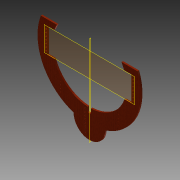
# Autodesk Inventor part: gyroYoke01_resized01
Saved by Autodesk Inventor 2013 (Build 170138000, 138)
## iProperties
Created: 2013-02-24
Part Number: gyroYoke01_resized01
Material: Wood (Oak)
Document SubType Name: Modeling
Designer: Nano
Density: 0.56 g/cm^3
Mass: 146.727 g
Surface Area: 937.732 cm^2
Volume: 262.012 cm^3
d0: 0.125 in
d1: 1.000 in
d3: 0.250 in
d4: 0.00 deg
d5: 0.250 in
d6: 0.250 in
d7: 0.250 in
d8: 0.250 in
d9: 0.125 in
d10: 0.125 in
d11: 0.250 in
d13: 0.250 in
d14: 0.00 deg
d15: 0.125 in
d22: 6.000 ul
d24: 0.500 in
d26: 0.00 deg
d27: 0.125 in
d34: 6.000 ul
d36: 0.500 in
d12: 0.250 in
Author: Nano
Autodesk Inventor part; units mm, degrees
ref_plane "YZ Plane" through (0, 0, 0) normal (1, 0, 0) x (0, 1, 0)
ref_plane "XZ Plane" through (0, 0, 0) normal (0, 1, 0) x (-1, 0, 0)
ref_plane "XY Plane" through (0, 0, 0) normal (0, 0, 1) x (1, 0, 0)
ref_plane "Work Plane1" through (0, 0, 0) normal (0, 0, 1) x (1, 0, 0)
sketch "Sketch1" plane through (0, 0, 0) normal (0, 0, 1) x (1, 0, 0)
  circle A0 centre (166.6875, 44.45) radius 6.35 construction
  line L0 (0, 0) -> (333.375, 0) construction
  line L1 (333.375, 0) -> (333.375, 88.9) construction
  line L2 (0, 88.9) -> (333.375, 88.9) construction
  line L3 (0, 0) -> (0, 88.9) construction
  line L4 (336.55, 95.25) -> (336.55, -6.35)
  line L5 (-3.175, -6.35) -> (-3.175, 95.25)
  arc A1 (361.952, -28.5758) -> (361.6406, 118.3031) centre (166.6875, 44.45) ccw
  arc A2 (109.447, -157.0949) -> (223.6431, -156.0919) centre (166.5241, -154.21) ccw
  arc A3 (223.6431, -156.0919) -> (230.1571, -154.1264) centre (166.6875, 44.45) ccw
  arc A4 (-29.5537, -28.941) -> (103.1936, -155.2131) centre (166.6875, 44.45) ccw
  arc A5 (-29.5402, 117.8769) -> (-29.5537, -28.941) centre (166.6875, 44.45) ccw
  arc A6 (336.55, 165.3087) -> (333.375, 169.6513) centre (166.6875, 44.45) ccw
  arc A7 (0, 169.6513) -> (-3.175, 165.3087) centre (166.6875, 44.45) ccw
  line L6 (361.6406, 118.3031) -> (296.5092, 118.3031)
  line L7 (35.5855, 117.8769) -> (-29.5402, 117.8769)
  arc A8 (194.8672, -103.8723) -> (308.8598, -6.35) centre (166.6875, 44.45) ccw
  arc A9 (307.1415, 95.25) -> (296.5092, 118.3031) centre (166.6875, 44.45) ccw
  arc A10 (35.5855, 117.8769) -> (25.271, 95.25) centre (166.6875, 44.45) ccw
  arc A11 (24.5152, -6.35) -> (136.5493, -103.4867) centre (166.6875, 44.45) ccw
  line L8 (-3.175, 95.25) -> (25.271, 95.25)
  line L9 (307.1415, 95.25) -> (336.55, 95.25)
  line L10 (336.55, -6.35) -> (308.8598, -6.35)
  line L11 (24.5152, -6.35) -> (-3.175, -6.35)
  line L12 (173.0375, -106.3919) -> (173.0375, -125.2673)
  line L13 (173.0375, -125.2673) -> (160.3375, -125.2673)
  line L14 (160.3375, -125.2673) -> (160.3375, -106.3919)
  line L15 (163.5125, -117.9837) -> (169.8625, -117.9837) projected
  line L16 (166.6875, 44.45) -> (38.9307, -83.3068) projected
  arc A12 (136.5493, -103.4867) -> (160.3375, -106.3919) centre (166.6875, 44.45) ccw
  arc A13 (173.0375, -106.3919) -> (194.8672, -103.8723) centre (166.6875, 44.45) ccw
  arc A14 (230.1571, -154.1264) -> (103.1936, -155.2131) centre (166.6875, -156.0919) ccw
  arc A15 (230.1571, -154.1264) -> (361.952, -28.5758) centre (166.6875, 44.45) ccw
  arc A16 (103.1936, -155.2131) -> (109.447, -157.0949) centre (166.6875, 44.45) ccw
  arc A17 (103.1936, -155.2131) -> (230.1571, -154.1264) centre (166.6875, -156.0919) ccw
  point P0 (166.6875, -117.9837)
  dimension "d0" = 3.175
  dimension "d5" = 6.35
  dimension "d6" = 6.35
  dimension "d7" = 6.35
  dimension "d8" = 6.35
  dimension "d9" = 3.175
  dimension "d10" = 3.175
  dimension "d11" = 6.35
  dimension "d12" = 6.35
  dimension "d47" = 127
  constraints: 34 point on circle, 22 end point, 17 centre point, 4 point on line, 1 coincident, 1 parallel, 1 other
  measures "d0" distance between parallel lines of L4 L1
  measures "d5" distance between parallel lines of L2 L9
  measures "d6" distance between parallel lines of L0 L10
  measures "d7" distance between parallel lines of L2 L8
  measures "d8" distance between parallel lines of L0 L11
  measures "d9" distance from line of L14 L15.start
  measures "d10" distance from line of L15.end L12
  measures "d11" distance from line of L12 point (166.688, -117.984)
  measures "d12" distance from line of point (166.688, -117.984) L14
  measures "d47" diameter of A14
extrude "Extrusion1" add sketch "Sketch1" against normal blind 6.35 contours L9 A9 L6 A1 A15 A14 A8 L10 L4 | A14 A3 A2 A16 A11 A12 L14 L13 L12 A13 A8 | A17 A16 A2 A3 | A14 A4 A5 L7 A10 L8 L5 L11 A11
sketch "Sketch2" plane through (0, 0, 0) normal (0, 0, 1) x (1, 0, 0)
  line L0 (339.725, 79.375) -> (346.075, 79.375) projected
  line L1 (346.075, 85.725) -> (346.075, 79.375) projected
  line L2 (346.075, 85.725) -> (339.725, 85.725) projected
  line L3 (339.725, 85.725) -> (339.725, 79.375) projected
  line L4 (339.725, 66.675) -> (346.075, 66.675) projected
  line L5 (346.075, 73.025) -> (346.075, 66.675) projected
  line L6 (346.075, 73.025) -> (339.725, 73.025) projected
  line L7 (339.725, 73.025) -> (339.725, 66.675) projected
  line L8 (339.725, 53.975) -> (346.075, 53.975) projected
  line L9 (346.075, 60.325) -> (346.075, 53.975) projected
  line L10 (346.075, 60.325) -> (339.725, 60.325) projected
  line L11 (339.725, 60.325) -> (339.725, 53.975) projected
  line L12 (346.075, 47.625) -> (339.725, 47.625) projected
  line L13 (339.725, 47.625) -> (339.725, 41.275) projected
  line L14 (339.725, 41.275) -> (346.075, 41.275) projected
  line L15 (346.075, 47.625) -> (346.075, 41.275) projected
  line L16 (346.075, 34.925) -> (339.725, 34.925) projected
  line L17 (339.725, 34.925) -> (339.725, 28.575) projected
  line L18 (339.725, 28.575) -> (346.075, 28.575) projected
  line L19 (346.075, 34.925) -> (346.075, 28.575) projected
  line L20 (346.075, 22.225) -> (339.725, 22.225) projected
  line L21 (339.725, 22.225) -> (339.725, 15.875) projected
  line L22 (339.725, 15.875) -> (346.075, 15.875) projected
  line L23 (346.075, 22.225) -> (346.075, 15.875) projected
  line L24 (346.075, 9.525) -> (339.725, 9.525) projected
  line L25 (339.725, 9.525) -> (339.725, 3.175) projected
  line L26 (339.725, 3.175) -> (346.075, 3.175) projected
  line L27 (346.075, 9.525) -> (346.075, 3.175) projected
  point P0 (0, 0)
extrude "Extrusion2" cut sketch "Sketch2" against normal blind 6.35
sketch "Sketch3" plane through (0, 0, 0) normal (0, 0, 1) x (1, 0, 0)
  line L0 (339.725, 15.875) -> (346.075, 9.525) construction
  line L1 (346.075, 15.875) -> (339.725, 9.525) construction
  point P0 (0, 0)
  point P1 (342.9, 12.7)
  constraints: 4 end point
hole "Hole1" at (342.9, 12.7, 0) direction (0, 0, -1) diameter 3.175 end through all
pattern_linear "Rectangular Pattern1" count 6 spacing 12.7 along (0, 1, 0) of "Hole1"
ref_plane "Work Plane2" through (166.6875, -125.2673, 0) normal (1, 0, 0) x (0, 0, -1)
mirror "Mirror1" about plane through (166.6875, -125.2673, 0) normal (1, 0, 0) of "Extrusion2", "Hole1", "Rectangular Pattern1"
sketch "Sketch5" plane through (0, 0, 0) normal (0, 0, 1) x (1, 0, 0)
  line L0 (150.8125, -110.6581) -> (147.6375, -110.6581)
  line L1 (147.6375, -110.6581) -> (147.6375, -116.7384)
  line L2 (147.6375, -116.7384) -> (150.8125, -116.7384)
  line L3 (150.8125, -110.6581) -> (150.8125, -116.7384)
  line L4 (147.6375, -129.4384) -> (150.8125, -129.4384)
  line L5 (150.8125, -123.0884) -> (150.8125, -129.4384)
  line L6 (150.8125, -123.0884) -> (147.6375, -123.0884)
  line L7 (147.6375, -123.0884) -> (147.6375, -129.4384)
  line L8 (150.8125, -135.7884) -> (147.6375, -135.7884)
  line L9 (147.6375, -135.7884) -> (147.6375, -142.1384)
  line L10 (147.6375, -142.1384) -> (150.8125, -142.1384)
  line L11 (150.8125, -135.7884) -> (150.8125, -142.1384)
  line L12 (147.6375, -154.8384) -> (150.8125, -154.8384)
  line L13 (150.8125, -148.4884) -> (150.8125, -154.8384)
  line L14 (150.8125, -148.4884) -> (147.6375, -148.4884)
  line L15 (147.6375, -148.4884) -> (147.6375, -154.8384)
  line L16 (150.8125, -161.1884) -> (147.6375, -161.1884)
  line L17 (147.6375, -161.1884) -> (147.6375, -167.5384)
  line L18 (147.6375, -167.5384) -> (150.8125, -167.5384)
  line L19 (150.8125, -161.1884) -> (150.8125, -167.5384)
  line L20 (147.6375, -180.2384) -> (150.8125, -180.2384)
  line L21 (150.8125, -173.8884) -> (150.8125, -180.2384)
  line L22 (150.8125, -173.8884) -> (147.6375, -173.8884)
  line L23 (147.6375, -173.8884) -> (147.6375, -180.2384)
  line L24 (150.8125, -186.5884) -> (147.6375, -186.5884)
  line L25 (147.6375, -186.5884) -> (147.6375, -202.4634)
  line L26 (147.6375, -202.4634) -> (150.8125, -202.4634)
  line L27 (150.8125, -186.5884) -> (150.8125, -202.4634)
  point P0 (0, 0)
extrude "Extrusion3" cut sketch "Sketch5" against normal through all
sketch "Sketch6" plane through (0, 0, 0) normal (0, 0, 1) x (1, 0, 0)
  line L0 (150.8125, -173.8884) -> (150.8125, -180.2384) construction
  line L1 (150.8125, -180.2384) -> (147.6375, -180.2384) construction
  line L2 (147.6375, -180.2384) -> (147.6375, -173.8884) construction
  line L3 (147.6375, -173.8884) -> (150.8125, -173.8884) construction
  line L4 (150.8125, -148.4884) -> (150.8125, -154.8384) construction
  line L5 (150.8125, -154.8384) -> (147.6375, -154.8384) construction
  line L6 (147.6375, -154.8384) -> (147.6375, -148.4884) construction
  line L7 (147.6375, -148.4884) -> (150.8125, -148.4884) construction
  line L8 (150.8125, -123.0884) -> (150.8125, -129.4384) construction
  line L9 (150.8125, -129.4384) -> (147.6375, -129.4384) construction
  line L10 (147.6375, -129.4384) -> (147.6375, -123.0884) construction
  line L11 (147.6375, -123.0884) -> (150.8125, -123.0884) construction
  line L12 (147.6375, -116.7384) -> (147.6375, -110.6581) construction
  line L13 (147.6375, -110.6581) -> (150.8125, -110.6581) construction
  line L14 (150.8125, -110.6581) -> (150.8125, -116.7384) construction
  line L15 (150.8125, -116.7384) -> (147.6375, -116.7384) construction
  line L16 (147.6375, -142.1384) -> (147.6375, -135.7884) construction
  line L17 (147.6375, -135.7884) -> (150.8125, -135.7884) construction
  line L18 (150.8125, -135.7884) -> (150.8125, -142.1384) construction
  line L19 (150.8125, -142.1384) -> (147.6375, -142.1384) construction
  line L20 (147.6375, -167.5384) -> (147.6375, -161.1884) construction
  line L21 (147.6375, -161.1884) -> (150.8125, -161.1884) construction
  line L22 (150.8125, -161.1884) -> (150.8125, -167.5384) construction
  line L23 (150.8125, -167.5384) -> (147.6375, -167.5384) construction
  line L24 (147.6375, -202.4634) -> (147.6375, -186.5884) construction
  line L25 (147.6375, -186.5884) -> (150.8125, -186.5884) construction
  line L26 (150.8125, -186.5884) -> (150.8125, -202.4634) construction
  line L27 (150.8125, -202.4634) -> (147.6375, -202.4634) construction
  circle A0 centre (-9.525, 76.2) radius 1.5875 construction
  circle A1 centre (-9.525, 63.5) radius 1.5875 construction
  circle A2 centre (-9.525, 50.8) radius 1.5875 construction
  circle A3 centre (-9.525, 38.1) radius 1.5875 construction
  circle A4 centre (-9.525, 25.4) radius 1.5875 construction
  line L28 (-6.35, 9.525) -> (-6.35, 3.175) construction
  line L29 (-6.35, 3.175) -> (-12.7, 3.175) construction
  line L30 (-12.7, 3.175) -> (-12.7, 9.525) construction
  line L31 (-12.7, 9.525) -> (-6.35, 9.525) construction
  line L32 (-6.35, 34.925) -> (-6.35, 28.575) construction
  line L33 (-6.35, 28.575) -> (-12.7, 28.575) construction
  line L34 (-12.7, 28.575) -> (-12.7, 34.925) construction
  line L35 (-12.7, 34.925) -> (-6.35, 34.925) construction
  line L36 (-12.7, 53.975) -> (-12.7, 60.325) construction
  line L37 (-12.7, 60.325) -> (-6.35, 60.325) construction
  line L38 (-6.35, 60.325) -> (-6.35, 53.975) construction
  line L39 (-6.35, 53.975) -> (-12.7, 53.975) construction
  line L40 (-12.7, 79.375) -> (-12.7, 85.725) construction
  line L41 (-12.7, 85.725) -> (-6.35, 85.725) construction
  line L42 (-6.35, 85.725) -> (-6.35, 79.375) construction
  line L43 (-6.35, 79.375) -> (-12.7, 79.375) construction
  line L44 (-12.7, 66.675) -> (-12.7, 73.025) construction
  line L45 (-12.7, 73.025) -> (-6.35, 73.025) construction
  line L46 (-6.35, 73.025) -> (-6.35, 66.675) construction
  line L47 (-6.35, 66.675) -> (-12.7, 66.675) construction
  line L48 (-6.35, 47.625) -> (-6.35, 41.275) construction
  line L49 (-6.35, 41.275) -> (-12.7, 41.275) construction
  line L50 (-12.7, 41.275) -> (-12.7, 47.625) construction
  line L51 (-12.7, 47.625) -> (-6.35, 47.625) construction
  line L52 (-6.35, 22.225) -> (-6.35, 15.875) construction
  line L53 (-6.35, 15.875) -> (-12.7, 15.875) construction
  line L54 (-12.7, 15.875) -> (-12.7, 22.225) construction
  line L55 (-12.7, 22.225) -> (-6.35, 22.225) construction
  circle A5 centre (-9.525, 12.7) radius 1.5875 construction
  circle A6 centre (342.9, 76.2) radius 1.5875 construction
  circle A7 centre (342.9, 63.5) radius 1.5875 construction
  circle A8 centre (342.9, 50.8) radius 1.5875 construction
  circle A9 centre (342.9, 38.1) radius 1.5875 construction
  circle A10 centre (342.9, 25.4) radius 1.5875 construction
  circle A11 centre (342.9, 12.7) radius 1.5875 construction
  line L56 (339.725, 15.875) -> (339.725, 22.225) construction
  line L57 (339.725, 22.225) -> (346.075, 22.225) construction
  line L58 (346.075, 22.225) -> (346.075, 15.875) construction
  line L59 (346.075, 15.875) -> (339.725, 15.875) construction
  line L60 (339.725, 41.275) -> (339.725, 47.625) construction
  line L61 (339.725, 47.625) -> (346.075, 47.625) construction
  line L62 (346.075, 47.625) -> (346.075, 41.275) construction
  line L63 (346.075, 41.275) -> (339.725, 41.275) construction
  line L64 (346.075, 73.025) -> (346.075, 66.675) construction
  line L65 (346.075, 66.675) -> (339.725, 66.675) construction
  line L66 (339.725, 66.675) -> (339.725, 73.025) construction
  line L67 (339.725, 73.025) -> (346.075, 73.025) construction
  line L68 (346.075, 85.725) -> (346.075, 79.375) construction
  line L69 (346.075, 79.375) -> (339.725, 79.375) construction
  line L70 (339.725, 79.375) -> (339.725, 85.725) construction
  line L71 (339.725, 85.725) -> (346.075, 85.725) construction
  line L72 (346.075, 60.325) -> (346.075, 53.975) construction
  line L73 (346.075, 53.975) -> (339.725, 53.975) construction
  line L74 (339.725, 53.975) -> (339.725, 60.325) construction
  line L75 (339.725, 60.325) -> (346.075, 60.325) construction
  line L76 (339.725, 28.575) -> (339.725, 34.925) construction
  line L77 (339.725, 34.925) -> (346.075, 34.925) construction
  line L78 (346.075, 34.925) -> (346.075, 28.575) construction
  line L79 (346.075, 28.575) -> (339.725, 28.575) construction
  line L80 (339.725, 3.175) -> (339.725, 9.525) construction
  line L81 (339.725, 9.525) -> (346.075, 9.525) construction
  line L82 (346.075, 9.525) -> (346.075, 3.175) construction
  line L83 (346.075, 3.175) -> (339.725, 3.175) construction
  line L84 (336.55, 95.25) -> (336.55, -6.35) construction
  line L85 (336.55, -6.35) -> (308.8598, -6.35) construction
  arc A12 (173.0375, -106.3919) -> (308.8598, -6.35) centre (166.6875, 44.45) ccw construction
  line L86 (173.0375, -106.3919) -> (173.0375, -125.2673) construction
  line L87 (173.0375, -125.2673) -> (160.3375, -125.2673) construction
  line L88 (160.3375, -125.2673) -> (160.3375, -106.3919) construction
  arc A13 (24.5152, -6.35) -> (160.3375, -106.3919) centre (166.6875, 44.45) ccw construction
  line L89 (24.5152, -6.35) -> (-3.175, -6.35) construction
  line L90 (-3.175, -6.35) -> (-3.175, 95.25) construction
  line L91 (-3.175, 95.25) -> (25.271, 95.25) construction
  arc A14 (35.5855, 117.8769) -> (25.271, 95.25) centre (166.6875, 44.45) ccw construction
  line L92 (35.5855, 117.8769) -> (-29.5402, 117.8769) construction
  arc A15 (-29.5402, 117.8769) -> (103.1936, -155.2131) centre (166.6875, 44.45) ccw construction
  arc A16 (230.1571, -154.1264) -> (361.6406, 118.3031) centre (166.6875, 44.45) ccw construction
  line L93 (361.6406, 118.3031) -> (296.5092, 118.3031) construction
  arc A17 (307.1415, 95.25) -> (296.5092, 118.3031) centre (166.6875, 44.45) ccw construction
  line L94 (307.1415, 95.25) -> (336.55, 95.25) construction
  line L95 (147.6375, -180.2384) -> (150.8125, -186.5884) construction
  line L96 (147.6375, -186.5884) -> (150.8125, -180.2384) construction
  arc A18 (103.1936, -155.2131) -> (230.1571, -154.1264) centre (166.6875, -156.0919) ccw projected
  point P0 (0, 0)
  point P1 (149.225, -183.4134)
  constraints: 4 end point
hole "Hole2" at (149.225, -183.4134, 0) direction (0, 0, -1) diameter 3.175 end through all
pattern_linear "Rectangular Pattern2" count 6 spacing 12.7 along (0, 1, 0) of "Hole2"
sketch "Sketch7" plane through (0, 0, 0) normal (0, 0, 1) x (1, 0, 0)
  point P0 (0, 0)
  point P1 (50.8818, -72.2337)
hole "Hole3" at (50.8818, -72.2337, 0) direction (0, 0, -1) diameter 3.175 end through all
pattern_linear "Rectangular Pattern3" count 4 spacing 12.7 along (0, -1, 0) of "Hole3"
mirror "Mirror2" about plane through (166.6875, -125.2673, 0) normal (1, 0, 0) of "Hole3", "Rectangular Pattern3"
equation "\"d6\" = d5"
equation "\"d7\" = d5"
equation "\"d8\" = d5"
equation "\"d10\" = d9"
body "Solid1"
